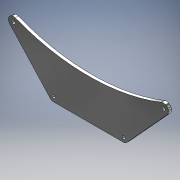
# Autodesk Inventor part: ハンド_下側板
Saved by Autodesk Inventor 2019.4 (Build 234330000, 330)
## iProperties
Created: 2021-12-05
Part Number: ハンド_下側板
Material: アルミニウム 6061
Document SubType Name: Modeling
Designer: 堀川皓史
Density: 2.7 g/cm^3
Appearance: アルミニウム - フラット
Author: 堀川皓史
Autodesk Inventor part; units mm, degrees
ref_plane "YZ Plane" through (0, 0, 0) normal (1, 0, 0) x (0, 1, 0)
ref_plane "XZ Plane" through (0, 0, 0) normal (0, 1, 0) x (-1, 0, 0)
ref_plane "XY Plane" through (0, 0, 0) normal (0, 0, 1) x (1, 0, 0)
sketch "スケッチ1" plane through (0, 0, 0) normal (0, 0, 1) x (1, 0, 0)
  circle A0 centre (-35, 0) radius 1.6
  circle A1 centre (35, 0) radius 1.6
  circle A2 centre (-75, 44.5) radius 1.6
  circle A3 centre (75, 44.5) radius 1.6
  arc A4 (-73.1707, 49.1534) -> (-78.6905, 41.1265) centre (-75, 44.5) ccw
  arc A5 (-38.3214, -3.0361) -> (-35, -4.5) centre (-35, 0) ccw
  arc A6 (35, -4.5) -> (38.3214, -3.0361) centre (35, 0) ccw
  arc A7 (78.6905, 41.1265) -> (73.1707, 49.1534) centre (75, 44.5) ccw
  arc A8 (-73.1707, 49.1534) -> (73.1707, 49.1534) centre (0, 235.2878) ccw
  line L0 (-78.6905, 41.1265) -> (-38.3214, -3.0361)
  line L1 (-35, -4.5) -> (35, -4.5)
  line L2 (38.3214, -3.0361) -> (78.6905, 41.1265)
  point P0 (0, 0)
  dimension "d0" = 3.2
  dimension "d1" = 3.2
  dimension "d2" = 70
  dimension "d3" = 35
  dimension "d4" = 3.2
  dimension "d5" = 3.2
  dimension "d6" = 44.5
  dimension "d7" = 150
  dimension "d8" = 75
  dimension "d9" = 5
  dimension "d10" = 4.5
  dimension "d11" = 4.5
  dimension "d12" = 5
  dimension "d13" = 200
  constraints: 10 point on circle, 9 centre point, 7 tangent, 6 end point, 4 coincident, 3 horizontal alignment, 1 horizontal
  measures "d0" diameter of A0
  measures "d1" diameter of A1
  measures "d2" distance of A1.centre A0.centre
  measures "d3" distance of point (0, 0) A0.centre
  measures "d4" diameter of A2
  measures "d5" diameter of A3
  measures "d6" vertical distance of A0.centre A2.centre
  measures "d7" distance of A3.centre A2.centre
  measures "d8" horizontal distance of point (0, 0) A2.centre
  measures "d9" radius of A4
  measures "d10" radius of A5
  measures "d11" radius of A6
  measures "d12" radius of A7
  measures "d13" radius of A8
extrude "押し出し1" add sketch "スケッチ1" along normal blind 3
equation "\"d3\" = 0.5 * d2"
equation "\"d8\" = 0.5 * d7"
